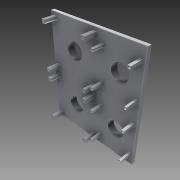
# Autodesk Inventor part: cameraPCBholder
Saved by Autodesk Inventor 2015 (Build 190159000, 159)
## iProperties
Created: 2015-03-20
Part Number: cameraPCBholder
Material: Aluminum 6061
Document SubType Name: Modeling
Designer: Akovo_000
Density: 2.7 g/cm^3
Appearance: Aluminum - Flat
Mass: 35.5834 g
Surface Area: 130.658 cm^2
Volume: 13.1791 cm^3
Author: Akovo_000
Autodesk Inventor part; units mm, degrees
ref_plane "YZ Plane" through (0, 0, 0) normal (1, 0, 0) x (0, 1, 0)
ref_plane "XZ Plane" through (0, 0, 0) normal (0, 1, 0) x (-1, 0, 0)
ref_plane "Main Work Pane" through (0, 2.75, 7) normal (0, 1, 0) x (-1, 0, 0)
sketch "Panel" plane through (0, 2.75, 7) normal (0, 1, 0) x (-1, 0, 0)
  line L0 (-5.834544, 44.988333) -> (60.165456, 44.988333)
  line L1 (20.965456, 12.982044) -> (-4.634544, 12.982044)
  line L2 (-4.634544, 12.982044) -> (-4.634544, 38.582044)
  line L3 (-4.634544, 38.582044) -> (20.965456, 38.582044)
  line L4 (20.965456, 38.582044) -> (20.965456, 12.982044)
  circle A0 centre (8.165452, 25.782047) radius 5.8
  line L5 (60.165456, -31.411667) -> (-5.834544, -31.411667)
  line L6 (20.965456, -25.015371) -> (-4.634544, -25.015371)
  line L7 (-4.634544, -25.015371) -> (-4.634544, 0.584629)
  line L8 (-4.634544, 0.584629) -> (20.965456, 0.584629)
  line L9 (20.965456, 0.584629) -> (20.965456, -25.015371)
  circle A1 centre (8.165456, -12.215371) radius 5.8
  line L10 (-5.834544, -31.411667) -> (-5.834544, 44.988333)
  line L11 (22.965456, 5.788333) -> (58.965456, 5.788333)
  line L12 (58.965456, 5.788333) -> (58.965456, -30.211667)
  line L13 (58.965456, -30.211667) -> (22.965456, -30.211667)
  line L14 (22.965456, -30.211667) -> (22.965456, 5.788333)
  line L15 (58.965456, 7.788333) -> (22.965456, 7.788333)
  line L16 (22.965456, 7.788333) -> (22.965456, 43.788333)
  line L17 (22.965456, 43.788333) -> (58.965456, 43.788333)
  line L18 (58.965456, 43.788333) -> (58.965456, 7.788333)
  line L19 (60.165456, -31.411667) -> (60.165456, 44.988333)
  circle A2 centre (40.965456, -12.211667) radius 5.8
  circle A3 centre (40.982778, 25.788333) radius 5.8
  line L20 (40.965456, -30.211667) -> (40.965456, -18.011667)
  line L21 (46.765456, -12.211668) -> (58.965456, -12.211667)
  line L22 (40.965456, -6.411667) -> (40.965456, 5.788333)
  line L23 (35.165456, -12.211668) -> (22.965456, -12.211667)
  line L24 (13.965456, -12.215371) -> (20.965456, -12.215371)
  line L25 (8.165456, -18.015371) -> (8.165456, -25.015371)
  line L26 (8.165456, -6.415371) -> (8.165456, 0.584629)
  line L27 (2.365456, -12.215371) -> (-4.634544, -12.215371)
  line L28 (8.165456, 19.982047) -> (8.165456, 12.982044)
  line L29 (13.965452, 25.782044) -> (20.965456, 25.782044)
  line L30 (8.172192, 31.582043) -> (8.165456, 38.582044)
  line L31 (2.365456, 25.78878) -> (-4.634544, 25.782044)
  line L32 (40.977196, 31.58833) -> (40.965456, 43.788333)
  line L33 (35.182778, 25.788333) -> (22.965456, 25.788333)
  line L34 (40.977196, 19.988336) -> (40.965456, 7.788333)
  line L35 (46.782778, 25.788333) -> (58.965456, 25.788333)
  point P0 (22.180169, 8.935201)
  point P1 (-5.819831, 8.726074)
  dimension "d317" = 25.6
  dimension "d318" = 25.6
  dimension "d319" = 25.6
  dimension "d320" = 25.6
  dimension "d321" = 36
  dimension "d322" = 36
  dimension "d323" = 36
  dimension "d324" = 36
  dimension "d325" = 2
  dimension "d326" = 1.2
  dimension "d327" = 1.2
  dimension "d328" = 1.2
  dimension "d329" = 1.2
  dimension "d330" = 2
  dimension "d331" = 2
  dimension "d333" = 1.2
  dimension "d334" = 1.2
  dimension "d337" = 11.6
  constraints: 73 end point, 16 midpoint, 15 point on circle, 10 equal length, 10 perpendicular, 8 parallel, 5 horizontal, 4 centre point, 4 line through centre, 3 equal radius, 3 vertical, 2 point on line
  measures "d317" distance between parallel lines of L3 L1
  measures "d318" distance between parallel lines of L8 L6
  measures "d319" distance between parallel lines of L2 L4
  measures "d320" distance between parallel lines of L9 L7
  measures "d321" distance of L12.end L13.end
  measures "d322" distance of L11.end L12.end
  measures "d323" distance of L16.end L17.end
  measures "d324" distance of L15.end L16.end
  measures "d325" distance between parallel lines of L15 L11
  measures "d326" distance between parallel lines of L13 L5
  measures "d327" distance between parallel lines of L0 L17
  measures "d328" distance between parallel lines of L10 L7
  measures "d329" distance between parallel lines of L10 L2
  measures "d330" distance between parallel lines of L14 L9
  measures "d331" distance between parallel lines of L16 L4
  measures "d333" distance between parallel lines of L19 L12
  measures "d334" distance between parallel lines of L19 L18
  measures "d337" diameter of A2
extrude "MainPanel" add sketch "Panel" along normal blind 2.5 contours L0 L19 L5 L10 | L1 L28 A0 L29 L4 | L1 L2 L31 A0 L28 | L29 A0 L30 L3 L4 | L2 L3 L30 A0 L31 | L6 L25 A1 L24 L9 | L6 L7 L27 A1 L25 | L24 A1 L26 L8 L9 | L7 L8 L26 A1 L27 | L11 L22 A2 L23 L14 | L11 L12 L21 A2 L22 | L23 A2 L20 L13 L14 | L12 L13 L20 A2 L21 | L15 L34 A3 L35 L18 | L15 L16 L33 A3 L34 | L35 A3 L32 L17 L18 | L16 L17 L32 A3 L33
sketch "BoardSuport" plane through (0, 2.75, 7) normal (0, -1, 0) x (1, 0, 0)
  line L0 (-19.415456, -23.465371) -> (3.084544, -23.465371)
  line L1 (3.084544, -23.465371) -> (3.084544, -0.965371)
  line L2 (3.084544, -0.965371) -> (-19.415456, -0.965371)
  line L3 (-19.415456, -0.965371) -> (-19.415456, -23.465371)
  circle A0 centre (-8.165456, -12.215371) radius 5.8
  line L4 (-19.415456, -23.465371) -> (3.084544, -0.965371) construction
  line L5 (3.084544, -23.465371) -> (-19.415456, -0.965371) construction
  circle A1 centre (-19.415456, -0.965371) radius 0.8
  circle A2 centre (3.084544, -0.965371) radius 0.8
  circle A3 centre (3.084544, -23.465371) radius 0.8
  circle A4 centre (-19.415456, -23.465371) radius 0.8
  circle A5 centre (-19.415456, -0.965371) radius 0.95
  circle A6 centre (3.084544, -0.965371) radius 0.95
  circle A7 centre (3.084544, -23.465371) radius 0.95
  circle A8 centre (-19.415456, -23.465371) radius 0.95
  line L6 (4.034544, -1.915371) -> (4.034544, -0.015371)
  line L7 (4.034544, -0.015371) -> (2.134544, -0.015371)
  line L8 (1.834544, -2.215371) -> (4.034544, -0.015371) construction
  line L9 (4.034544, -1.915371) -> (2.134544, -0.015371) construction
  line L10 (2.134544, -0.015371) -> (2.134544, -0.965371)
  line L11 (4.034544, -1.915371) -> (3.084544, -1.915371)
  line L12 (4.034544, -22.515371) -> (4.034544, -24.415371)
  line L13 (4.034544, -24.415371) -> (2.134544, -24.415371)
  line L14 (1.984544, -22.365371) -> (4.034544, -24.415371) construction
  line L15 (4.034544, -22.515371) -> (2.134544, -24.415371) construction
  line L16 (4.034544, -22.515371) -> (3.084544, -22.515371)
  line L17 (2.134544, -24.415371) -> (2.134544, -23.465371)
  line L18 (-56.465456, -27.711667) -> (-25.465456, -27.711667)
  line L19 (-25.465456, -27.711667) -> (-25.465456, 3.288333)
  line L20 (-25.465456, 3.288333) -> (-56.465456, 3.288333)
  line L21 (-56.465456, 3.288333) -> (-56.465456, -27.711667)
  circle A9 centre (-40.965456, -12.211667) radius 5.8
  line L22 (-56.465456, -27.711667) -> (-25.465456, 3.288333) construction
  line L23 (-25.465456, -27.711667) -> (-56.465456, 3.288333) construction
  line L24 (-56.482778, 10.288333) -> (-25.482778, 10.288333)
  line L25 (-25.482778, 10.288333) -> (-25.482778, 41.288333)
  line L26 (-25.482778, 41.288333) -> (-56.482778, 41.288333)
  line L27 (-56.482778, 41.288333) -> (-56.482778, 10.288333)
  circle A10 centre (-40.982778, 25.788333) radius 5.8
  line L28 (-56.482778, 10.288333) -> (-25.482778, 41.288333) construction
  line L29 (-25.482778, 10.288333) -> (-56.482778, 41.288333) construction
  line L30 (-19.415456, 14.538333) -> (3.084544, 14.538333)
  line L31 (3.084544, 14.538333) -> (3.084544, 37.038333)
  line L32 (3.084544, 37.038333) -> (-19.415456, 37.038333)
  line L33 (-19.415456, 37.038333) -> (-19.415456, 14.538333)
  line L34 (-19.415456, 14.538333) -> (3.084544, 37.038333) construction
  line L35 (3.084544, 14.538333) -> (-19.415456, 37.038333) construction
  circle A11 centre (-19.415456, 37.038333) radius 0.8
  circle A12 centre (3.084544, 37.038333) radius 0.8
  circle A13 centre (3.084544, 14.538333) radius 0.8
  circle A14 centre (-19.415456, 14.538333) radius 0.8
  circle A15 centre (-19.415456, 14.538333) radius 0.95
  circle A16 centre (-19.415456, 37.038333) radius 0.95
  circle A17 centre (3.084544, 37.038333) radius 0.95
  circle A18 centre (3.084544, 14.538333) radius 0.95
  line L36 (-18.465456, 13.588333) -> (-20.365456, 13.588333)
  line L37 (-20.365456, 13.588333) -> (-20.365456, 15.488333)
  line L38 (-20.365456, 15.488333) -> (-18.465456, 13.588333) construction
  line L39 (-18.465456, 15.488333) -> (-20.365456, 13.588333) construction
  line L40 (-20.365456, 37.988333) -> (-18.465456, 37.988333)
  line L41 (-20.365456, 36.088333) -> (-20.365456, 37.988333)
  line L42 (-20.365456, 37.988333) -> (-18.465456, 36.088333) construction
  line L43 (-18.465456, 37.988333) -> (-20.365456, 36.088333) construction
  line L44 (2.134544, 37.988333) -> (4.034544, 37.988333)
  line L45 (4.034544, 37.988333) -> (4.034544, 36.088333)
  line L46 (2.134544, 37.988333) -> (4.034544, 36.088333) construction
  line L47 (4.034544, 37.988333) -> (2.134544, 36.088333) construction
  line L48 (4.034544, 15.488333) -> (4.034544, 13.588333)
  line L49 (4.034544, 13.588333) -> (2.134544, 13.588333)
  line L50 (2.134544, 15.488333) -> (4.034544, 13.588333) construction
  line L51 (4.034544, 15.488333) -> (2.134544, 13.588333) construction
  line L52 (-19.415456, 15.488333) -> (-20.365456, 15.488333)
  line L53 (-18.465456, 13.588333) -> (-18.465456, 14.538333)
  line L54 (-18.465456, 37.988333) -> (-18.465456, 37.038333)
  line L55 (-20.365456, 36.088333) -> (-19.415456, 36.088333)
  line L56 (2.134544, 37.988333) -> (2.134544, 37.038333)
  line L57 (4.034544, 36.088333) -> (3.084544, 36.088333)
  line L58 (2.134544, 14.538333) -> (2.134544, 13.588333)
  line L59 (3.084544, 15.488333) -> (4.034544, 15.488333)
  circle A19 centre (-25.482778, 41.288333) radius 0.8
  circle A20 centre (-25.482778, 41.288333) radius 1.4
  circle A21 centre (-25.482778, 10.288333) radius 0.8
  circle A22 centre (-25.482778, 10.288333) radius 1.4
  circle A23 centre (-56.482778, 10.288333) radius 0.8
  circle A24 centre (-56.482778, 10.288333) radius 1.4
  circle A25 centre (-56.482778, 41.288333) radius 0.8
  circle A26 centre (-56.482778, 41.288333) radius 1.4
  circle A27 centre (-56.465456, 3.288333) radius 0.8
  circle A28 centre (-25.465456, 3.288333) radius 0.8
  circle A29 centre (-25.465456, 3.288333) radius 1.4
  circle A30 centre (-56.465456, 3.288333) radius 1.4
  circle A31 centre (-56.465456, -27.711667) radius 0.8
  circle A32 centre (-56.465456, -27.711667) radius 1.4
  circle A33 centre (-25.465456, -27.711667) radius 0.8
  circle A34 centre (-25.465456, -27.711667) radius 1.4
  line L60 (-55.064034, -29.110243) -> (-57.864033, -29.113089)
  line L61 (-57.864033, -29.113089) -> (-57.866877, -26.31309)
  line L62 (-57.866877, -26.31309) -> (-55.064034, -29.110243) construction
  line L63 (-54.867083, -26.110042) -> (-57.864033, -29.113089) construction
  line L64 (-24.066275, -26.310849) -> (-24.064637, -29.110848)
  line L65 (-24.064637, -29.110848) -> (-26.864637, -29.112485)
  line L66 (-27.066391, -26.112603) -> (-24.064637, -29.110848) construction
  line L67 (-24.066275, -26.310849) -> (-26.864637, -29.112485) construction
  line L68 (-26.882778, 4.705655) -> (-24.082778, 4.705655)
  line L69 (-24.082778, 4.705655) -> (-24.082778, 1.905655)
  line L70 (-26.882778, 4.705655) -> (-24.082778, 1.905655) construction
  line L71 (-24.082778, 4.705655) -> (-27.045433, 1.668769) construction
  line L72 (-57.965456, 4.788333) -> (-54.965456, 1.788333) construction
  line L73 (-54.965456, 4.788333) -> (-57.965456, 1.788333) construction
  line L74 (-55.082778, 8.888333) -> (-57.882778, 8.888333)
  line L75 (-57.882778, 8.888333) -> (-57.882778, 11.688333)
  line L76 (-57.882778, 11.688333) -> (-55.082778, 8.888333) construction
  line L77 (-54.882778, 11.888333) -> (-57.882778, 8.888333) construction
  line L78 (-24.082778, 11.688333) -> (-24.082778, 8.888333)
  line L79 (-24.082778, 8.888333) -> (-26.882778, 8.888333)
  line L80 (-27.000099, 11.805655) -> (-24.082778, 8.888333) construction
  line L81 (-24.082778, 11.688333) -> (-26.882778, 8.888333) construction
  line L82 (-57.882778, 42.688333) -> (-55.082778, 42.688333)
  line L83 (-57.882778, 39.888333) -> (-57.882778, 42.688333)
  line L84 (-57.882778, 42.688333) -> (-54.882778, 39.688333) construction
  line L85 (-55.082778, 42.688333) -> (-57.882778, 39.888333) construction
  line L86 (-55.064034, -29.110243) -> (-55.065456, -27.711667)
  line L87 (-57.866877, -26.31309) -> (-56.465456, -26.311667)
  line L88 (-24.066275, -26.310849) -> (-25.465456, -26.311667)
  line L89 (-26.864637, -29.112485) -> (-26.865456, -27.711667)
  line L90 (-57.865456, 4.688333) -> (-55.065456, 4.688333)
  line L91 (-57.865456, 1.888333) -> (-57.865456, 4.688333)
  line L92 (-57.865456, 4.688333) -> (-54.965456, 1.788333) construction
  line L93 (-55.065456, 4.688333) -> (-57.865456, 1.888333) construction
  line L94 (-57.865456, 1.888333) -> (-56.465456, 1.888333)
  line L95 (-55.065456, 4.688333) -> (-55.065456, 3.288333)
  line L96 (-24.082778, 11.688333) -> (-25.482778, 11.688333)
  line L97 (-24.082778, 1.905655) -> (-25.465456, 1.888333)
  line L98 (-26.882778, 4.705655) -> (-26.865456, 3.288333)
  line L99 (-55.082778, 8.888333) -> (-55.082778, 10.288333)
  line L100 (-57.882778, 11.688333) -> (-56.482778, 11.688333)
  line L101 (-26.882778, 8.888333) -> (-26.882778, 10.288333)
  line L102 (-55.082778, 42.688333) -> (-55.082778, 41.288333)
  line L103 (-57.882778, 39.888333) -> (-56.482778, 39.888333)
  line L104 (-26.882778, 42.688333) -> (-24.082778, 42.688333)
  line L105 (-24.082778, 42.688333) -> (-24.082778, 39.888333)
  line L106 (-26.882778, 42.688333) -> (-24.082778, 39.888333) construction
  line L107 (-24.082778, 42.688333) -> (-26.882778, 39.888333) construction
  line L108 (-26.882778, 42.688333) -> (-26.882778, 41.288333)
  line L109 (-24.082778, 39.888333) -> (-25.482778, 39.888333)
  line L110 (-18.465456, -24.415371) -> (-20.365456, -24.415371)
  line L111 (-20.365456, -24.415371) -> (-20.365456, -22.515371)
  line L112 (-20.365456, -22.515371) -> (-18.465456, -24.415371) construction
  line L113 (-18.465456, -22.515371) -> (-20.365456, -24.415371) construction
  line L114 (-19.415456, -22.515371) -> (-20.365456, -22.515371)
  line L115 (-18.465456, -23.465371) -> (-18.465456, -24.415371)
  line L116 (-20.365456, -0.015371) -> (-18.465456, -0.015371)
  line L117 (-20.365456, -1.915371) -> (-20.365456, -0.015371)
  line L118 (-20.365456, -0.015371) -> (-18.465456, -1.915371) construction
  line L119 (-18.465456, -0.015371) -> (-20.365456, -1.915371) construction
  line L120 (-18.465456, -0.015371) -> (-18.465456, -0.965371)
  line L121 (-20.365456, -1.915371) -> (-19.415456, -1.915371)
  point P0 (-8.165456, 25.788333)
  dimension "d435" = 22.5
  dimension "d436" = 1.6
  dimension "d451" = 22.5
  dimension "d452" = 22.5
  dimension "d456" = 1.6
  dimension "d457" = 1.9
  dimension "d458" = 1.9
  dimension "d459" = 2.8
  dimension "d460" = 1.6
  dimension "d462" = 31
  dimension "d463" = 31
  dimension "d464" = 31
  dimension "d465" = 31
  constraints: 244 end point, 50 point on line, 32 coincident, 32 midpoint, 31 centre point, 30 point on circle, 22 tangent, 20 equal length, 19 equal radius, 14 perpendicular, 13 horizontal, 8 parallel, 1 horizontal alignment, 9 other
  measures "d435" distance of L1.end L0.end
  measures "d436" diameter of A1
  measures "d451" distance of L32.end L31.end
  measures "d452" distance of L31.end L30.end
  measures "d456" diameter of A14
  measures "d457" diameter of A15
  measures "d458" diameter of A5
  measures "d459" diameter of A32
  measures "d460" diameter of A31
  measures "d462" distance between parallel lines of L24 L26
  measures "d463" distance between parallel lines of L25 L27
  measures "d464" distance between parallel lines of L18 L20
  measures "d465" distance between parallel lines of L19 L21
sketch "LensHolders" plane through (0, 5.25, 7) normal (0, 1, 0) x (1, 0, 0)
  circle A0 centre (-40.982778, -25.788333) radius 5.8
  circle A1 centre (-40.982778, -25.788333) radius 5.8
  circle A2 centre (-40.982778, -25.788333) radius 8.3
  circle A3 centre (-8.165452, -25.782047) radius 5.8
  circle A4 centre (-8.165452, -25.782047) radius 5.8
  circle A5 centre (-8.165452, -25.782047) radius 8.2
  circle A6 centre (-40.965456, 12.211667) radius 5.8
  circle A7 centre (-40.965456, 12.211667) radius 5.8
  circle A8 centre (-40.965456, 12.211667) radius 8.2
  circle A9 centre (-8.165456, 12.215371) radius 5.8
  circle A10 centre (-8.165456, 12.215371) radius 5.8
  circle A11 centre (-8.165456, 12.215371) radius 8.849954
  dimension "d369" = 0
  dimension "d370" = 0
  dimension "d371" = 0
  dimension "d372" = 2.5
  dimension "d373" = 0
  dimension "d374" = 0
  dimension "d377" = 0
  dimension "d378" = 0
  dimension "d381" = 0
  dimension "d382" = 0
  constraints: 8 centre point, 4 coincident, 3 equal radius
  measures "d369" distance of A0.centre A1.centre
  measures "d370" distance of A1.centre A0.centre
  measures "d371" radial gap between concentric circles of A1 A0
  measures "d372" radial gap between concentric circles of A2 A0
  measures "d373" distance of A3.centre A4.centre
  measures "d374" distance of A4.centre A3.centre
  measures "d377" distance of A6.centre A7.centre
  measures "d378" distance of A7.centre A6.centre
  measures "d381" distance of A9.centre A10.centre
  measures "d382" distance of A9.centre A10.centre
extrude "LensHolder" add sketch "LensHolders" along normal blind 2.5
thread "Thread9" size "M12x0.5" class "6H" standard "ANSI Metric M Profile" full length
thread "Thread10" size "M12x0.5" class "6H" standard "ANSI Metric M Profile" full length
thread "Thread11" size "M12x0.5" class "6H" standard "ANSI Metric M Profile" full length
thread "Thread12" size "M12x0.5" class "6H" standard "ANSI Metric M Profile" full length
sketch "BoardSuport outline for Extrusion11" plane through (0, 2.75, 7) normal (0, -1, 0) x (1, 0, 0)
  arc A0 (2.134544, 37.038333) -> (3.084544, 36.088333) centre (3.084544, 37.038333) ccw
  line L0 (3.084544, 36.088333) -> (4.034544, 36.088333)
  line L1 (4.034544, 36.088333) -> (4.034544, 37.988333)
  line L2 (4.034544, 37.988333) -> (2.134544, 37.988333)
  line L3 (2.134544, 37.988333) -> (2.134544, 37.038333)
  arc A1 (-19.415456, 36.088333) -> (-18.465456, 37.038333) centre (-19.415456, 37.038333) ccw
  line L4 (-18.465456, 37.038333) -> (-18.465456, 37.988333)
  line L5 (-18.465456, 37.988333) -> (-20.365456, 37.988333)
  line L6 (-20.365456, 37.988333) -> (-20.365456, 36.088333)
  line L7 (-20.365456, 36.088333) -> (-19.415456, 36.088333)
  arc A2 (-18.465456, 14.538333) -> (-19.415456, 15.488333) centre (-19.415456, 14.538333) ccw
  line L8 (-19.415456, 15.488333) -> (-20.365456, 15.488333)
  line L9 (-20.365456, 15.488333) -> (-20.365456, 13.588333)
  line L10 (-20.365456, 13.588333) -> (-18.465456, 13.588333)
  line L11 (-18.465456, 13.588333) -> (-18.465456, 14.538333)
  arc A3 (3.084544, 15.488333) -> (2.134544, 14.538333) centre (3.084544, 14.538333) ccw
  line L12 (2.134544, 14.538333) -> (2.134544, 13.588333)
  line L13 (2.134544, 13.588333) -> (4.034544, 13.588333)
  line L14 (4.034544, 13.588333) -> (4.034544, 15.488333)
  line L15 (4.034544, 15.488333) -> (3.084544, 15.488333)
  arc A4 (-18.465456, -23.465371) -> (-19.415456, -22.515371) centre (-19.415456, -23.465371) ccw
  line L16 (-19.415456, -22.515371) -> (-20.365456, -22.515371)
  line L17 (-20.365456, -22.515371) -> (-20.365456, -24.415371)
  line L18 (-20.365456, -24.415371) -> (-18.465456, -24.415371)
  line L19 (-18.465456, -24.415371) -> (-18.465456, -23.465371)
  arc A5 (2.134544, -0.965371) -> (3.084544, -1.915371) centre (3.084544, -0.965371) ccw
  line L20 (3.084544, -1.915371) -> (4.034544, -1.915371)
  line L21 (4.034544, -1.915371) -> (4.034544, -0.015371)
  line L22 (4.034544, -0.015371) -> (2.134544, -0.015371)
  line L23 (2.134544, -0.015371) -> (2.134544, -0.965371)
  arc A6 (3.084544, -22.515371) -> (2.134544, -23.465371) centre (3.084544, -23.465371) ccw
  line L24 (2.134544, -23.465371) -> (2.134544, -24.415371)
  line L25 (2.134544, -24.415371) -> (4.034544, -24.415371)
  line L26 (4.034544, -24.415371) -> (4.034544, -22.515371)
  line L27 (4.034544, -22.515371) -> (3.084544, -22.515371)
  arc A7 (-26.865456, 3.288333) -> (-25.465456, 1.888333) centre (-25.465456, 3.288333) ccw
  line L28 (-25.465456, 1.888333) -> (-24.082778, 1.905655)
  line L29 (-24.082778, 1.905655) -> (-24.082778, 4.705655)
  line L30 (-24.082778, 4.705655) -> (-26.882778, 4.705655)
  line L31 (-26.882778, 4.705655) -> (-26.865456, 3.288333)
  arc A8 (-26.882778, 41.288333) -> (-25.482778, 39.888333) centre (-25.482778, 41.288333) ccw
  line L32 (-25.482778, 39.888333) -> (-24.082778, 39.888333)
  line L33 (-24.082778, 39.888333) -> (-24.082778, 42.688333)
  line L34 (-24.082778, 42.688333) -> (-26.882778, 42.688333)
  line L35 (-26.882778, 42.688333) -> (-26.882778, 41.288333)
  arc A9 (-55.065456, -27.711667) -> (-56.465456, -26.311667) centre (-56.465456, -27.711667) ccw
  line L36 (-56.465456, -26.311667) -> (-57.866877, -26.31309)
  line L37 (-57.866877, -26.31309) -> (-57.864033, -29.113089)
  line L38 (-57.864033, -29.113089) -> (-55.064034, -29.110243)
  line L39 (-55.064034, -29.110243) -> (-55.065456, -27.711667)
  arc A10 (-25.465456, -26.311667) -> (-26.865456, -27.711667) centre (-25.465456, -27.711667) ccw
  line L40 (-26.865456, -27.711667) -> (-26.864637, -29.112485)
  line L41 (-26.864637, -29.112485) -> (-24.064637, -29.110848)
  line L42 (-24.064637, -29.110848) -> (-24.066275, -26.310849)
  line L43 (-24.066275, -26.310849) -> (-25.465456, -26.311667)
  arc A11 (-56.482778, 39.888333) -> (-55.082778, 41.288333) centre (-56.482778, 41.288333) ccw
  line L44 (-55.082778, 41.288333) -> (-55.082778, 42.688333)
  line L45 (-55.082778, 42.688333) -> (-57.882778, 42.688333)
  line L46 (-57.882778, 42.688333) -> (-57.882778, 39.888333)
  line L47 (-57.882778, 39.888333) -> (-56.482778, 39.888333)
  arc A12 (-55.082778, 10.288333) -> (-56.482778, 11.688333) centre (-56.482778, 10.288333) ccw
  line L48 (-56.482778, 11.688333) -> (-57.882778, 11.688333)
  line L49 (-57.882778, 11.688333) -> (-57.882778, 8.888333)
  line L50 (-57.882778, 8.888333) -> (-55.082778, 8.888333)
  line L51 (-55.082778, 8.888333) -> (-55.082778, 10.288333)
  arc A13 (-25.482778, 11.688333) -> (-26.882778, 10.288333) centre (-25.482778, 10.288333) ccw
  line L52 (-26.882778, 10.288333) -> (-26.882778, 8.888333)
  line L53 (-26.882778, 8.888333) -> (-24.082778, 8.888333)
  line L54 (-24.082778, 8.888333) -> (-24.082778, 11.688333)
  line L55 (-24.082778, 11.688333) -> (-25.482778, 11.688333)
  arc A14 (-19.415456, -1.915371) -> (-18.465456, -0.965371) centre (-19.415456, -0.965371) ccw
  line L56 (-18.465456, -0.965371) -> (-18.465456, -0.015371)
  line L57 (-18.465456, -0.015371) -> (-20.365456, -0.015371)
  line L58 (-20.365456, -0.015371) -> (-20.365456, -1.915371)
  line L59 (-20.365456, -1.915371) -> (-19.415456, -1.915371)
  line L60 (-57.865456, 1.888333) -> (-56.465456, 1.888333)
  arc A15 (-56.465456, 1.888333) -> (-55.065456, 3.288333) centre (-56.465456, 3.288333) ccw
  line L61 (-55.065456, 3.288333) -> (-55.065456, 4.688333)
  line L62 (-55.065456, 4.688333) -> (-57.865456, 4.688333)
  line L63 (-57.865456, 4.688333) -> (-57.865456, 1.888333)
extrude "Extrusion11" add sketch "BoardSuport outline for Extrusion11" along normal blind 8.5
sketch "Sketch16" plane through (0, -5.75, 7) normal (0, -1, 0) x (1, 0, 0)
  line L0 (-19.415456, -23.465371) -> (3.084544, -23.465371)
  line L1 (3.084544, -23.465371) -> (3.084544, -0.965371)
  line L2 (3.084544, -0.965371) -> (-19.415456, -0.965371)
  line L3 (-19.415456, -0.965371) -> (-19.415456, -23.465371)
  circle A0 centre (-8.165456, -12.215371) radius 5.8
  line L4 (-19.415456, -23.465371) -> (3.084544, -0.965371) construction
  line L5 (3.084544, -23.465371) -> (-19.415456, -0.965371) construction
  circle A1 centre (-19.415456, -0.965371) radius 0.8
  circle A2 centre (3.084544, -0.965371) radius 0.8
  circle A3 centre (3.084544, -23.465371) radius 0.8
  circle A4 centre (-19.415456, -23.465371) radius 0.8
  circle A5 centre (-19.415456, -0.965371) radius 0.95
  circle A6 centre (3.084544, -0.965371) radius 0.95
  circle A7 centre (3.084544, -23.465371) radius 0.95
  circle A8 centre (-19.415456, -23.465371) radius 0.95
  line L6 (4.034544, -1.915371) -> (4.034544, -0.015371)
  line L7 (4.034544, -0.015371) -> (2.134544, -0.015371)
  line L8 (1.834544, -2.215371) -> (4.034544, -0.015371) construction
  line L9 (4.034544, -1.915371) -> (2.134544, -0.015371) construction
  line L10 (2.134544, -0.015371) -> (2.134544, -0.965371)
  line L11 (4.034544, -1.915371) -> (3.084544, -1.915371)
  line L12 (4.034544, -22.515371) -> (4.034544, -24.415371)
  line L13 (4.034544, -24.415371) -> (2.134544, -24.415371)
  line L14 (1.984544, -22.365371) -> (4.034544, -24.415371) construction
  line L15 (4.034544, -22.515371) -> (2.134544, -24.415371) construction
  line L16 (4.034544, -22.515371) -> (3.084544, -22.515371)
  line L17 (2.134544, -24.415371) -> (2.134544, -23.465371)
  line L18 (-56.465456, -27.711667) -> (-25.465456, -27.711667)
  line L19 (-25.465456, -27.711667) -> (-25.465456, 3.288333)
  line L20 (-25.465456, 3.288333) -> (-56.465456, 3.288333)
  line L21 (-56.465456, 3.288333) -> (-56.465456, -27.711667)
  circle A9 centre (-40.965456, -12.211667) radius 5.8
  line L22 (-56.465456, -27.711667) -> (-25.465456, 3.288333) construction
  line L23 (-25.465456, -27.711667) -> (-56.465456, 3.288333) construction
  line L24 (-56.482778, 10.288333) -> (-25.482778, 10.288333)
  line L25 (-25.482778, 10.288333) -> (-25.482778, 41.288333)
  line L26 (-25.482778, 41.288333) -> (-56.482778, 41.288333)
  line L27 (-56.482778, 41.288333) -> (-56.482778, 10.288333)
  circle A10 centre (-40.982778, 25.788333) radius 5.8
  line L28 (-56.482778, 10.288333) -> (-25.482778, 41.288333) construction
  line L29 (-25.482778, 10.288333) -> (-56.482778, 41.288333) construction
  line L30 (-19.415456, 14.538333) -> (3.084544, 14.538333)
  line L31 (3.084544, 14.538333) -> (3.084544, 37.038333)
  line L32 (3.084544, 37.038333) -> (-19.415456, 37.038333)
  line L33 (-19.415456, 37.038333) -> (-19.415456, 14.538333)
  line L34 (-19.415456, 14.538333) -> (3.084544, 37.038333) construction
  line L35 (3.084544, 14.538333) -> (-19.415456, 37.038333) construction
  circle A11 centre (-19.415456, 37.038333) radius 0.8
  circle A12 centre (3.084544, 37.038333) radius 0.8
  circle A13 centre (3.084544, 14.538333) radius 0.8
  circle A14 centre (-19.415456, 14.538333) radius 0.8
  circle A15 centre (-19.415456, 14.538333) radius 0.95
  circle A16 centre (-19.415456, 37.038333) radius 0.95
  circle A17 centre (3.084544, 37.038333) radius 0.95
  circle A18 centre (3.084544, 14.538333) radius 0.95
  line L36 (-18.465456, 13.588333) -> (-20.365456, 13.588333)
  line L37 (-20.365456, 13.588333) -> (-20.365456, 15.488333)
  line L38 (-20.365456, 15.488333) -> (-18.465456, 13.588333) construction
  line L39 (-18.465456, 15.488333) -> (-20.365456, 13.588333) construction
  line L40 (-20.365456, 37.988333) -> (-18.465456, 37.988333)
  line L41 (-20.365456, 36.088333) -> (-20.365456, 37.988333)
  line L42 (-20.365456, 37.988333) -> (-18.465456, 36.088333) construction
  line L43 (-18.465456, 37.988333) -> (-20.365456, 36.088333) construction
  line L44 (2.134544, 37.988333) -> (4.034544, 37.988333)
  line L45 (4.034544, 37.988333) -> (4.034544, 36.088333)
  line L46 (2.134544, 37.988333) -> (4.034544, 36.088333) construction
  line L47 (4.034544, 37.988333) -> (2.134544, 36.088333) construction
  line L48 (4.034544, 15.488333) -> (4.034544, 13.588333)
  line L49 (4.034544, 13.588333) -> (2.134544, 13.588333)
  line L50 (2.134544, 15.488333) -> (4.034544, 13.588333) construction
  line L51 (4.034544, 15.488333) -> (2.134544, 13.588333) construction
  line L52 (-19.415456, 15.488333) -> (-20.365456, 15.488333)
  line L53 (-18.465456, 13.588333) -> (-18.465456, 14.538333)
  line L54 (-18.465456, 37.988333) -> (-18.465456, 37.038333)
  line L55 (-20.365456, 36.088333) -> (-19.415456, 36.088333)
  line L56 (2.134544, 37.988333) -> (2.134544, 37.038333)
  line L57 (4.034544, 36.088333) -> (3.084544, 36.088333)
  line L58 (2.134544, 14.538333) -> (2.134544, 13.588333)
  line L59 (3.084544, 15.488333) -> (4.034544, 15.488333)
  circle A19 centre (-25.482778, 41.288333) radius 0.8
  circle A20 centre (-25.482778, 41.288333) radius 1.4
  circle A21 centre (-25.482778, 10.288333) radius 0.8
  circle A22 centre (-25.482778, 10.288333) radius 1.4
  circle A23 centre (-56.482778, 10.288333) radius 0.8
  circle A24 centre (-56.482778, 10.288333) radius 1.4
  circle A25 centre (-56.482778, 41.288333) radius 0.8
  circle A26 centre (-56.482778, 41.288333) radius 1.4
  circle A27 centre (-56.465456, 3.288333) radius 0.8
  circle A28 centre (-25.465456, 3.288333) radius 0.8
  circle A29 centre (-25.465456, 3.288333) radius 1.4
  circle A30 centre (-56.465456, 3.288333) radius 1.4
  circle A31 centre (-56.465456, -27.711667) radius 0.8
  circle A32 centre (-56.465456, -27.711667) radius 1.4
  circle A33 centre (-25.465456, -27.711667) radius 0.8
  circle A34 centre (-25.465456, -27.711667) radius 1.4
  line L60 (-55.064034, -29.110243) -> (-57.864033, -29.113089)
  line L61 (-57.864033, -29.113089) -> (-57.866877, -26.31309)
  line L62 (-57.866877, -26.31309) -> (-55.064034, -29.110243) construction
  line L63 (-54.867083, -26.110042) -> (-57.864033, -29.113089) construction
  line L64 (-24.066275, -26.310849) -> (-24.064637, -29.110848)
  line L65 (-24.064637, -29.110848) -> (-26.864637, -29.112485)
  line L66 (-27.066391, -26.112603) -> (-24.064637, -29.110848) construction
  line L67 (-24.066275, -26.310849) -> (-26.864637, -29.112485) construction
  line L68 (-26.882778, 4.705655) -> (-24.082778, 4.705655)
  line L69 (-24.082778, 4.705655) -> (-24.082778, 1.905655)
  line L70 (-26.882778, 4.705655) -> (-24.082778, 1.905655) construction
  line L71 (-24.082778, 4.705655) -> (-27.045433, 1.668769) construction
  line L72 (-57.965456, 4.788333) -> (-54.965456, 1.788333) construction
  line L73 (-54.965456, 4.788333) -> (-57.965456, 1.788333) construction
  line L74 (-55.082778, 8.888333) -> (-57.882778, 8.888333)
  line L75 (-57.882778, 8.888333) -> (-57.882778, 11.688333)
  line L76 (-57.882778, 11.688333) -> (-55.082778, 8.888333) construction
  line L77 (-54.882778, 11.888333) -> (-57.882778, 8.888333) construction
  line L78 (-24.082778, 11.688333) -> (-24.082778, 8.888333)
  line L79 (-24.082778, 8.888333) -> (-26.882778, 8.888333)
  line L80 (-27.000099, 11.805655) -> (-24.082778, 8.888333) construction
  line L81 (-24.082778, 11.688333) -> (-26.882778, 8.888333) construction
  line L82 (-57.882778, 42.688333) -> (-55.082778, 42.688333)
  line L83 (-57.882778, 39.888333) -> (-57.882778, 42.688333)
  line L84 (-57.882778, 42.688333) -> (-54.882778, 39.688333) construction
  line L85 (-55.082778, 42.688333) -> (-57.882778, 39.888333) construction
  line L86 (-55.064034, -29.110243) -> (-55.065456, -27.711667)
  line L87 (-57.866877, -26.31309) -> (-56.465456, -26.311667)
  line L88 (-24.066275, -26.310849) -> (-25.465456, -26.311667)
  line L89 (-26.864637, -29.112485) -> (-26.865456, -27.711667)
  line L90 (-57.865456, 4.688333) -> (-55.065456, 4.688333)
  line L91 (-57.865456, 1.888333) -> (-57.865456, 4.688333)
  line L92 (-57.865456, 4.688333) -> (-54.965456, 1.788333) construction
  line L93 (-55.065456, 4.688333) -> (-57.865456, 1.888333) construction
  line L94 (-57.865456, 1.888333) -> (-56.465456, 1.888333)
  line L95 (-55.065456, 4.688333) -> (-55.065456, 3.288333)
  line L96 (-24.082778, 11.688333) -> (-25.482778, 11.688333)
  line L97 (-24.082778, 1.905655) -> (-25.465456, 1.888333)
  line L98 (-26.882778, 4.705655) -> (-26.865456, 3.288333)
  line L99 (-55.082778, 8.888333) -> (-55.082778, 10.288333)
  line L100 (-57.882778, 11.688333) -> (-56.482778, 11.688333)
  line L101 (-26.882778, 8.888333) -> (-26.882778, 10.288333)
  line L102 (-55.082778, 42.688333) -> (-55.082778, 41.288333)
  line L103 (-57.882778, 39.888333) -> (-56.482778, 39.888333)
  line L104 (-26.882778, 42.688333) -> (-24.082778, 42.688333)
  line L105 (-24.082778, 42.688333) -> (-24.082778, 39.888333)
  line L106 (-26.882778, 42.688333) -> (-24.082778, 39.888333) construction
  line L107 (-24.082778, 42.688333) -> (-26.882778, 39.888333) construction
  line L108 (-26.882778, 42.688333) -> (-26.882778, 41.288333)
  line L109 (-24.082778, 39.888333) -> (-25.482778, 39.888333)
  line L110 (-18.465456, -24.415371) -> (-20.365456, -24.415371)
  line L111 (-20.365456, -24.415371) -> (-20.365456, -22.515371)
  line L112 (-20.365456, -22.515371) -> (-18.465456, -24.415371) construction
  line L113 (-18.465456, -22.515371) -> (-20.365456, -24.415371) construction
  line L114 (-19.415456, -22.515371) -> (-20.365456, -22.515371)
  line L115 (-18.465456, -23.465371) -> (-18.465456, -24.415371)
  line L116 (-20.365456, -0.015371) -> (-18.465456, -0.015371)
  line L117 (-20.365456, -1.915371) -> (-20.365456, -0.015371)
  line L118 (-20.365456, -0.015371) -> (-18.465456, -1.915371) construction
  line L119 (-18.465456, -0.015371) -> (-20.365456, -1.915371) construction
  line L120 (-18.465456, -0.015371) -> (-18.465456, -0.965371)
  line L121 (-20.365456, -1.915371) -> (-19.415456, -1.915371)
  point P0 (0, -7)
  point P1 (-8.165456, 25.788333)
  dimension "d470" = 22.5
  dimension "d471" = 1.6
  dimension "d472" = 22.5
  dimension "d473" = 22.5
  dimension "d474" = 1.6
  dimension "d475" = 1.9
  dimension "d476" = 1.9
  dimension "d477" = 2.8
  dimension "d478" = 1.6
  dimension "d479" = 31
  dimension "d480" = 31
  dimension "d481" = 31
  dimension "d482" = 31
  constraints: 244 end point, 50 point on line, 34 centre point, 32 coincident, 32 midpoint, 30 point on circle, 22 tangent, 20 equal length, 19 equal radius, 14 perpendicular, 13 horizontal, 8 parallel, 1 horizontal alignment, 9 other
  measures "d470" distance of L1.end L0.end
  measures "d471" diameter of A1
  measures "d472" distance of L32.end L31.end
  measures "d473" distance of L31.end L30.end
  measures "d474" diameter of A14
  measures "d475" diameter of A15
  measures "d476" diameter of A5
  measures "d477" diameter of A32
  measures "d478" diameter of A31
  measures "d479" distance between parallel lines of L24 L26
  measures "d480" distance between parallel lines of L25 L27
  measures "d481" distance between parallel lines of L18 L20
  measures "d482" distance between parallel lines of L19 L21
hole "Hole6" at (-25.465456, -5.75, 10.288333) at (-19.415456, -5.75, 6.034629) at (-19.415456, -5.75, -16.465371) at (-25.465456, -5.75, -20.711667) at (3.084544, -5.75, 6.034629) at (3.084544, -5.75, -16.465371) at (3.084544, -5.75, 21.538333) at (3.084544, -5.75, 44.038333) at (-19.415456, -5.75, 44.038333) at (-19.415456, -5.75, 21.538333) at (-25.482778, -5.75, 17.288333) at (-25.482778, -5.75, 48.288333) at (-56.482778, -5.75, 48.288333) at (-56.482778, -5.75, 17.288333) at (-56.465456, -5.75, 10.288333) at (-56.465456, -5.75, -20.711667) direction (0, 1, 0) diameter 1.6 depth 8 tip angle 118
body "Solid2"
